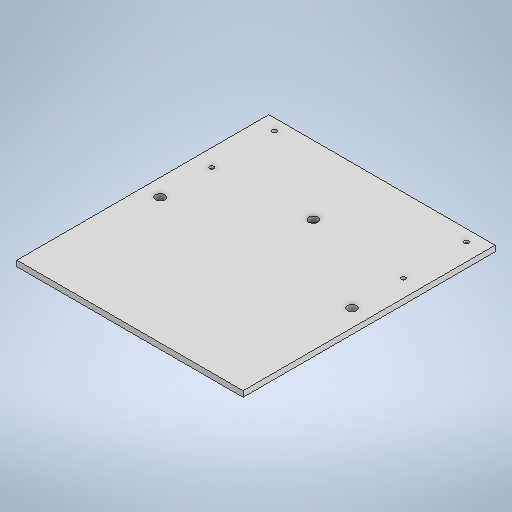
# Autodesk Inventor part: panel1
Saved by Autodesk Inventor 2025.3 (Build 293356000, 356)
## iProperties
Created: 2026-04-19
Part Number: panel1
Material: Generic
Document SubType Name: Modeling
Designer: ksawe
Density: 1 g/cm^3
Appearance: Default
Author: ksawe
Autodesk Inventor part; units mm, degrees
ref_plane "YZ Plane" through (0, 0, 0) normal (1, 0, 0) x (0, 1, 0)
ref_plane "XZ Plane" through (0, 0, 0) normal (0, 1, 0) x (-1, 0, 0)
ref_plane "XY Plane" through (0, 0, 0) normal (0, 0, 1) x (1, 0, 0)
sketch "Sketch1" plane through (0, 0, 0) normal (0, 1, 0) x (-1, 0, 0)
  line L0 (98.75, 110) -> (-98.75, 110)
  line L1 (-98.75, 110) -> (-98.75, -110)
  line L2 (-98.75, -110) -> (98.75, -110)
  line L3 (98.75, -110) -> (98.75, 110)
  line L4 (98.75, 110) -> (-98.75, -110) construction
  line L5 (-98.75, 110) -> (98.75, -110) construction
  circle A0 centre (-83.75, 0) radius 4
  line L6 (0, 110) -> (0, -110)
  circle A1 centre (83.75, 0) radius 4
  circle A2 centre (0, -50) radius 4
  point P0 (0, 0)
  point P1 (0, 0)
  dimension "d0" = 197.5
  dimension "d1" = 220
  dimension "d2" = 8
  dimension "d3" = 8
  dimension "d4" = 15
  dimension "d5" = 8
  dimension "d6" = 50
  dimension "d7" = 15
  constraints: 14 end point, 5 midpoint, 3 centre point, 2 horizontal alignment, 2 parallel, 1 horizontal, 1 perpendicular, 1 point on line, 1 vertical alignment
  measures "d0" distance of L0.start L0.end
  measures "d1" distance of L0.end L1.end
  measures "d2" diameter of A0
  measures "d3" diameter of A1
  measures "d4" distance from line of L1 A0.centre
  measures "d5" diameter of A2
  measures "d6" vertical distance of A1.centre A2.centre
  measures "d7" distance from line of L3 A1.centre
extrude "Extrusion1" add sketch "Sketch1" along normal blind 5 contours L3 L2 L6 A2 L0 | L6 A2 L2 L1 L0
sketch "Sketch2" plane through (0, 5, 0) normal (0, 1, 0) x (1, 0, 0)
  line L0 (-98.75, 110) -> (-98.75, -110) projected
  line L1 (98.75, -110) -> (98.75, 110) projected
  line L2 (98.75, 110) -> (-98.75, 110) projected
  point P0 (0, 0)
  point P1 (83.75, 45)
  point P2 (83.75, 100)
  point P3 (-83.75, 45)
  point P4 (-83.75, 100)
  dimension "d10" = 15
  dimension "d11" = 15
  dimension "d12" = 15
  dimension "d13" = 15
  dimension "d14" = 10
  dimension "d15" = 10
  dimension "d23" = 65
  dimension "d24" = 65
  measures "d10" distance from line of L0 point (-83.75, 45)
  measures "d11" distance from line of L0 point (-83.75, 100)
  measures "d12" distance from line of L1 point (83.75, 45)
  measures "d13" distance from line of L1 point (83.75, 100)
  measures "d14" distance from line of L2 point (83.75, 100)
  measures "d15" distance from line of L2 point (-83.75, 100)
  measures "d23" distance from line of L2 point (-83.75, 45)
  measures "d24" distance from line of L2 point (83.75, 45)
hole "Hole1" at (83.75, 5, -100) at (-83.75, 5, -100) at (-83.75, 5, -45) at (83.75, 5, -45) direction (0, -1, 0) diameter 2 depth 4 tip angle 118 counterbore diameter 3.9 counterbore depth 2
body "Solid1"
